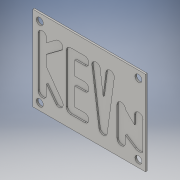
# Autodesk Inventor part: NamePlate
Saved by Autodesk Inventor 2016 (Build 200138000, 138)
## iProperties
Created: 2016-09-28
Part Number: NamePlate
Material: Generic
Document SubType Name: Modeling
Designer: Kevin
Density: 1 g/cm^3
Appearance: Default
Author: Kevin
Autodesk Inventor part; units mm, degrees
ref_plane "YZ Plane" through (0, 0, 0) normal (1, 0, 0) x (0, 1, 0)
ref_plane "XZ Plane" through (0, 0, 0) normal (0, 1, 0) x (-1, 0, 0)
ref_plane "XY Plane" through (0, 0, 0) normal (0, 0, 1) x (1, 0, 0)
sketch "Sketch1" plane through (0, 0, 0) normal (0, 0, 1) x (1, 0, 0)
  line L0 (0, 0) -> (203.2, 0)
  line L1 (203.2, 0) -> (203.2, -152.4)
  line L2 (203.2, -152.4) -> (0, -152.4)
  line L3 (0, -152.4) -> (0, 0)
  line L4 (0, 0) -> (12.7, 0)
  line L5 (0, -12.7) -> (0, 0)
  line L6 (0, -152.4) -> (0, -139.7)
  line L7 (203.2, 0) -> (190.5, 0)
  line L8 (203.2, -152.4) -> (203.2, -139.7)
  circle A0 centre (12.7, -12.7) radius 6.35
  circle A1 centre (190.5, -12.7) radius 6.35
  circle A2 centre (190.5, -139.7) radius 6.35
  circle A3 centre (12.7, -139.7) radius 6.35
  constraints: 18 end point, 4 centre point, 3 point on line, 2 horizontal, 2 parallel, 1 perpendicular
extrude "Extrusion1" add sketch "Sketch1" along normal blind 3.175
sketch "Sketch2" plane through (0, 0, 3.175) normal (0, 0, 1) x (1, 0, 0)
  arc A0 (24.817, -32.5655) -> (9.577, -32.5655) centre (17.197, -32.5655) ccw
  arc A1 (9.577, -122.0402) -> (24.817, -122.0402) centre (17.197, -122.0402) ccw
  line L0 (9.577, -32.5655) -> (9.577, -122.0402)
  line L1 (9.577, -42.2151) -> (9.577, -32.5655)
  arc A2 (53.0983, -37.3903) -> (42.7617, -26.7428) centre (46.6851, -33.275) ccw
  arc A3 (49.095, -40.7739) -> (42.7617, -26.7428) centre (46.7521, -33.3865) ccw
  line L2 (42.7617, -26.7428) -> (24.817, -40.0522)
  line L3 (53.0983, -37.3903) -> (24.3404, -58.7199)
  arc A4 (42.2851, -127.8629) -> (53.0983, -117.2154) centre (47.2004, -122.0402) ccw
  line L4 (53.0983, -117.2154) -> (24.3404, -77.3028)
  line L5 (42.2851, -127.8629) -> (24.817, -104.3113)
  line L6 (24.817, -104.3113) -> (24.817, -122.0402)
  line L7 (24.3404, -58.7199) -> (24.3404, -77.3028)
  line L8 (24.817, -40.0522) -> (24.817, -32.5655)
  line L9 (60.5227, -33.6636) -> (60.5227, -122.5636)
  line L10 (68.1427, -130.1836) -> (93.5427, -130.1836)
  line L11 (93.5427, -114.9436) -> (75.7627, -114.9436)
  line L12 (68.1427, -26.0436) -> (93.5427, -26.0436)
  line L13 (93.5427, -41.2836) -> (75.7627, -41.2836)
  arc A5 (68.1427, -26.0436) -> (60.5227, -33.6636) centre (68.1427, -33.6636) ccw
  arc A6 (60.5227, -122.5636) -> (68.1427, -130.1836) centre (68.1427, -122.5636) ccw
  arc A7 (93.5427, -130.1836) -> (93.5427, -114.9436) centre (93.5427, -122.5636) ccw
  arc A8 (93.5427, -41.2836) -> (93.5427, -26.0436) centre (93.5427, -33.6636) ccw
  arc A9 (93.5427, -81.8927) -> (93.5427, -66.6527) centre (93.5427, -74.2727) ccw
  line L14 (93.5427, -66.6527) -> (75.7627, -66.6527)
  line L15 (93.5427, -81.8927) -> (75.7627, -81.8927)
  line L16 (75.7627, -41.2836) -> (75.7627, -66.6527)
  line L17 (75.7627, -81.8927) -> (75.7627, -114.9436)
  line L18 (147.1171, -32.5701) -> (134.4171, -125.4887)
  line L19 (106.4768, -32.5655) -> (119.2541, -126.5682)
  line L20 (121.6953, -32.0671) -> (126.8219, -72.9902)
  line L21 (126.8219, -72.9902) -> (131.9604, -32.2167)
  arc A10 (147.1171, -32.5701) -> (131.9604, -32.2167) centre (139.5207, -33.1695) ccw
  arc A11 (119.2541, -126.5682) -> (134.4171, -125.4887) centre (126.801, -125.5424) ccw
  arc A12 (121.6953, -32.0671) -> (106.4768, -32.5655) centre (114.109, -33.0174) ccw
  line L22 (151.8189, -72.9902) -> (151.8189, -126.5682)
  arc A13 (167.0589, -72.9902) -> (151.8189, -72.9902) centre (159.4389, -72.9902) ccw
  arc A14 (151.8189, -125.6862) -> (167.0589, -126.5682) centre (159.4644, -125.6862) ccw
  line L23 (198.7066, -72.9518) -> (198.7066, -124.1784)
  line L24 (184.3126, -124.8116) -> (167.0589, -113.0447)
  line L25 (183.4405, -72.9518) -> (183.4405, -89.0244)
  line L26 (183.4405, -89.0244) -> (167.0589, -72.9902)
  line L27 (167.0589, -113.0447) -> (167.0589, -126.5682)
  arc A15 (198.7066, -72.9518) -> (183.4405, -72.9518) centre (191.0735, -72.9518) ccw
  arc A16 (184.3126, -124.8116) -> (198.7066, -124.1784) centre (191.0866, -114.8789) ccw
  point P0 (0, 0)
  constraints: 56 end point, 34 point on circle, 17 centre point, 17 tangent, 6 vertical, 4 parallel, 1 perpendicular, 1 point on line
emboss "Emboss1" sketch "Sketch2" operation cut depth 2.54 direction (0, 0, -1)
body "Solid1"
